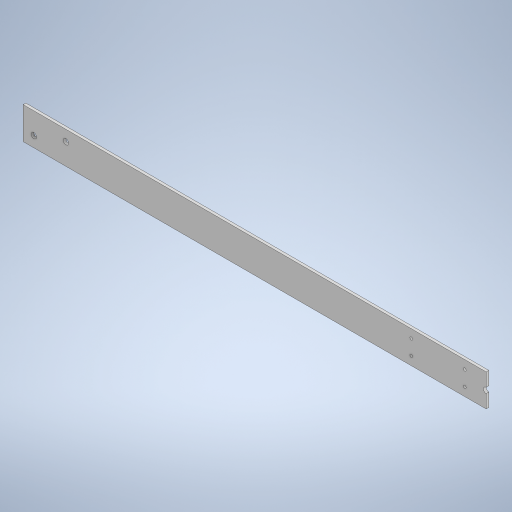
# Autodesk Inventor part: arm projectile
Saved by Autodesk Inventor 2023 (Build 270158000, 158)
## iProperties
Created: 2023-10-16
Part Number: arm projectile
Material: Generic
Document SubType Name: Modeling
Designer: Nate
Density: 1 g/cm^3
Appearance: Default
Author: Nate
Autodesk Inventor part; units mm, degrees
ref_plane "YZ Plane" through (0, 0, 0) normal (1, 0, 0) x (0, 1, 0)
ref_plane "XZ Plane" through (0, 0, 0) normal (0, 1, 0) x (-1, 0, 0)
ref_plane "XY Plane" through (0, 0, 0) normal (0, 0, 1) x (1, 0, 0)
sketch "Sketch1" plane through (0, 0, 0) normal (0, 0, 1) x (1, 0, 0)
  line L0 (0, 0) -> (-550.0116, 0)
  line L1 (-550.0116, 0) -> (-550.0116, 38.1)
  line L2 (-550.0116, 38.1) -> (0, 38.1)
  line L3 (0, 38.1) -> (0, 0)
  circle A0 centre (0, 19.05) radius 3.175
  circle A1 centre (-25.4, 10.16) radius 1.5875
  circle A2 centre (-25.4, 27.94) radius 1.5875
  circle A3 centre (-88.9, 27.94) radius 1.5875
  circle A4 centre (-88.9, 10.16) radius 1.5875
  circle A5 centre (-499.2116, 25.4) radius 3.175
  circle A6 centre (-537.3116, 12.7) radius 3.175
  point P0 (0, 15.875)
  point P1 (0, 22.225)
  dimension "d0" = 38.1
  dimension "d1" = 550.0116
  dimension "d2" = 6.35
  dimension "d3" = 3.175
  dimension "d4" = 3.175
  dimension "d5" = 3.175
  dimension "d6" = 3.175
  dimension "d7" = 10.16
  dimension "d8" = 10.16
  dimension "d9" = 10.16
  dimension "d10" = 10.16
  dimension "d11" = 25.4
  dimension "d12" = 25.4
  dimension "d13" = 88.9
  dimension "d14" = 88.9
  dimension "d15" = 6.35
  dimension "d16" = 6.35
  dimension "d18" = 50.8
  dimension "d19" = 12.7
  dimension "d23" = 12.7
  dimension "d24" = 12.7
  constraints: 8 end point, 7 centre point, 2 parallel, 1 horizontal, 1 midpoint, 1 perpendicular
  measures "d0" distance between parallel lines of L2 L0
  measures "d1" distance between parallel lines of L3 L1
  measures "d2" diameter of A0
  measures "d3" diameter of A1
  measures "d4" diameter of A2
  measures "d5" diameter of A3
  measures "d6" diameter of A4
  measures "d7" distance from line of L2 A3.centre
  measures "d8" distance from line of L2 A2.centre
  measures "d9" distance from line of L0 A1.centre
  measures "d10" distance from line of L0 A4.centre
  measures "d11" distance from line of L3 A1.centre
  measures "d12" distance from line of L3 A2.centre
  measures "d13" distance from line of L3 A3.centre
  measures "d14" distance from line of L3 A4.centre
  measures "d15" diameter of A6
  measures "d16" diameter of A5
  measures "d18" distance from line of L1 A5.centre
  measures "d19" distance from line of L1 A6.centre
  measures "d23" distance from line of L2 A5.centre
  measures "d24" distance from line of L0 A6.centre
extrude "Extrusion1" add sketch "Sketch1" along normal blind 3.175 contours L0 L1 L2 L3 A0
body "Solid1"
